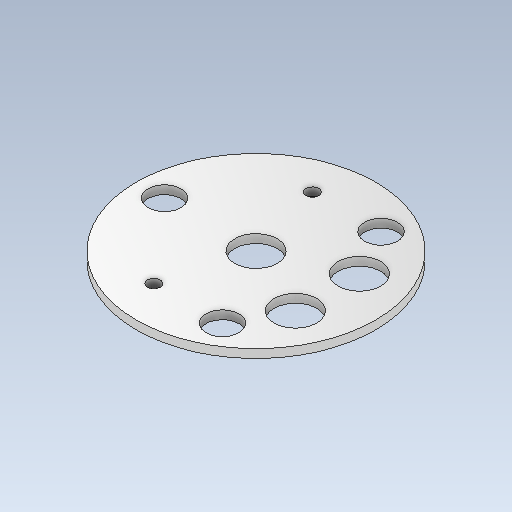
# Autodesk Inventor part: buffer
Saved by Autodesk Inventor 2020 (Build 240168000, 168)
## iProperties
Created: 2019-06-21
Part Number: buffer
Material: PBT Plastic
Document SubType Name: Modeling
Designer: ColinP
Density: 8 g/cm^3
Appearance: Clear - Light
Mass: 8.49189 g
Surface Area: 19.6339 cm^2
Volume: 1.06149 cm^3
Author: ColinP
Autodesk Inventor part; units mm, degrees
ref_plane "YZ Plane" through (0, 0, 0) normal (1, 0, 0) x (0, 1, 0)
ref_plane "XZ Plane" through (0, 0, 0) normal (0, 1, 0) x (-1, 0, 0)
ref_plane "XY Plane" through (0, 0, 0) normal (0, 0, 1) x (1, 0, 0)
sketch "Sketch1" plane through (0, 0, 0) normal (0, 1, 0) x (-1, 0, 0)
  circle A0 centre (0, 0) radius 17.78
  dimension "d0" = 35.56
  constraints: 1 centre point, 1 coincident
  measures "d0" diameter of A0
extrude "Extrusion1" add sketch "Sketch1" along normal blind 1.27
sketch "Sketch2" plane through (0, 1.27, 0) normal (0, 1, 0) x (1, 0, 0)
  circle A0 centre (0, 0) radius 17.78 projected
  constraints: 1 coincident
hole "Hole1" at (0, 1.27, 0) direction (0, -1, 0) diameter 6.35 end through all
sketch "Sketch3" plane through (0, 1.27, 0) normal (0, 1, 0) x (1, 0, 0)
  line L0 (0, 0) -> (-13.6144, 0)
  dimension "d10" = 13.6144
  constraints: 2 end point, 1 horizontal
  measures "d10" distance of L0.start L0.end
hole "Hole2" at (-13.6144, 1.27, 0) direction (0, -1, 0) diameter 4.9022 end through all
pattern_circular "Circular Pattern1" count 3 over 360 about axis through (0, -49.0355, 0) along (0, 1, 0) of "Hole2"
sketch "Sketch5" plane through (0, 1.27, 0) normal (0, 1, 0) x (1, 0, 0)
  circle A0 centre (-13.6144, 0) radius 2.4511 projected
  circle A1 centre (6.8072, 11.7904) radius 2.4511 projected
  line L0 (-13.6144, 0) -> (6.8072, 11.7904)
  circle A2 centre (6.8072, -11.7904) radius 2.4511 projected
  line L1 (6.8072, 11.7904) -> (6.8072, -11.7904)
  line L2 (6.8072, -11.7904) -> (-13.6144, 0)
  line L3 (-13.6144, 0) -> (-13.6144, -11.7904)
  line L4 (-13.6144, -11.7904) -> (6.8072, -11.7904)
  line L5 (-13.6144, 0) -> (-13.6144, 11.7904)
  line L6 (-13.6144, 11.7904) -> (6.8072, 11.7904)
  circle A3 centre (-3.4036, 11.7904) radius 0.635
  circle A4 centre (-3.4036, -11.7904) radius 0.635
  point P0 (0, 0)
  dimension "d28" = 1.27
  constraints: 14 end point, 2 centre point, 2 midpoint, 2 vertical, 1 perpendicular, 1 point on line
  measures "d28" diameter of A3
hole "Hole4" at (-3.4036, 1.27, 11.7904) at (-3.4036, 1.27, -11.7904) direction (0, -1, 0) diameter 1.905 depth 6.35 tip angle 118
sketch "Sketch6" plane through (0, 1.27, 0) normal (0, 1, 0) x (1, 0, 0)
  circle A0 centre (6.8072, 11.7904) radius 2.4511 projected
  circle A1 centre (6.8072, -11.7904) radius 2.4511 projected
  line L0 (6.8072, 11.7904) -> (6.8072, -11.7904)
  line L1 (0, 0) -> (17.6436, 0)
  line L2 (0, 0) -> (12.7, 0)
  line L3 (0, 0) -> (17.78, 0)
  circle A2 centre (0, 0) radius 17.78 projected
  line L4 (6.8072, 0) -> (10.6172, 0)
  line L5 (10.6172, 0) -> (10.6172, 6.35)
  line L6 (10.6172, 6.35) -> (10.6172, -6.35)
  line L7 (10.6172, -6.35) -> (10.6172, -3.175)
  line L8 (10.6172, -3.175) -> (10.6172, 3.175)
  line L9 (10.6172, 6.35) -> (10.6172, 3.175)
  line L10 (10.6172, -3.175) -> (10.6172, -6.35)
  circle A3 centre (10.6172, 4.7625) radius 3.175
  circle A4 centre (10.6172, -4.7625) radius 3.175
  dimension "d36" = 12.7
  dimension "d37" = 3.81
  dimension "d38" = 6.35
  dimension "d39" = 12.7
  dimension "d40" = 3.175
  dimension "d41" = 6.35
  dimension "d42" = 180
  dimension "d43" = 6.35
  dimension "d44" = 6.35
  constraints: 22 end point, 6 point on line, 3 midpoint, 2 centre point, 2 horizontal, 2 vertical, 1 collinear, 1 horizontal alignment, 1 perpendicular, 1 other
  measures "d36" distance of L1.start L2.end
  measures "d37" distance of L4.start L4.end
  measures "d38" distance of L4.end L5.end
  measures "d39" distance of L5.end L6.end
  measures "d40" distance of L6.end L7.end
  measures "d41" distance of L7.end L8.end
  measures "d42" angle of L8 L7
  measures "d43" diameter of A3
  measures "d44" diameter of A4
hole "Hole5" at (10.6172, 1.27, -4.7625) at (10.6172, 1.27, 4.7625) direction (0, -1, 0) diameter 6.35 depth 6.35
body "Solid1"
